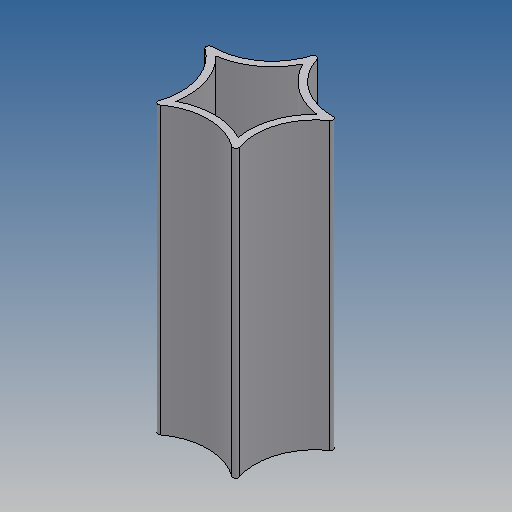
# Autodesk Inventor part: 21700_stern
Saved by Autodesk Inventor 2019.4 (Build 234330000, 330)
## iProperties
Part Number: 21700_stern
Material: GEDA Stahl
Document SubType Name: Modeling
Designer: Admin
Mass: 31.4795 g
Surface Area: 66.7703 cm^2
Volume: 4.00503 cm^3
Density: 7.86 g/cm^3
Appearance: GEDA Stahl A
Gewicht: 0,031 kg
G_L: 0
G_H: 0
G_B: 0
InventorVersion: 2019.4
VAULT_Status: in Bearbeitung
Revision: -
Max. Breite: 0
Max. Höhe: 0
Max. Länge: 0
Max. Abmessungen: 0 x 0 x 0
Volumen: 4005,026
Author: Admin
Autodesk Inventor part; units mm, degrees
note: some values were not read from the file. Left out: dimensions or parameters whose unit could not be read.
ref_plane "YZ Plane" through (0, 0, 0) normal (1, 0, 0) x (0, 1, 0)
ref_plane "XZ Plane" through (0, 0, 0) normal (0, 1, 0) x (-1, 0, 0)
ref_plane "XY Plane" through (0, 0, 0) normal (0, 0, 1) x (1, 0, 0)
sketch "Skizze1" plane through (0, 0, 0) normal (0, 0, 1) x (1, 0, 0)
  circle A0 centre (-10.5, 14.452) radius 10.5
  circle A1 centre (0, 0) radius 17.8637 construction
  circle A2 centre (10.5, 14.452) radius 10.5
  circle A3 centre (16.9894, -5.5202) radius 10.5
  circle A4 centre (0, -17.8637) radius 10.5
  circle A5 centre (-16.9894, -5.5202) radius 10.5
  arc A6 (-13.7447, 4.4659) -> (0, 14.452) centre (-10.5, 14.452) ccw
  arc A7 (0, 14.452) -> (13.7447, 4.4659) centre (10.5, 14.452) ccw
  arc A8 (13.7447, 4.4659) -> (8.4947, -11.6919) centre (16.9894, -5.5202) ccw
  arc A9 (8.4947, -11.6919) -> (-8.4947, -11.6919) centre (0, -17.8637) ccw
  arc A10 (-8.4947, -11.6919) -> (-13.7447, 4.4659) centre (-16.9894, -5.5202) ccw
  dimension "d0" = 21
  dimension "d1" = 10.5
  constraints: 15 point on circle, 13 equal radius, 11 centre point, 6 coincident, 1 vertical alignment
  measures "d0" diameter of A0
  measures "d1" radius of A7
extrude "Extrusion1" add sketch "Skizze1" along normal blind 50 contours A2 A3 A4 A5 A0
fillet "Rundung1" radius 0.5 5 edges at (0, 14.452, 25) (13.7447, 4.4659, 25) (-13.7447, 4.4659, 25) (-8.4947, -11.6919, 25) (8.4947, -11.6919, 25)
sketch "Skizze2" plane through (0, 0, 50) normal (0, 0, 1) x (1, 0, 0)
  arc A0 (6.269, -9.4405) -> (7.0412, -8.8794) centre (6.5675, -9.0394) ccw projected
  arc A1 (10.9157, 3.0449) -> (7.0412, -8.8794) centre (16.9894, -5.5202) ccw projected
  arc A2 (10.9157, 3.0449) -> (10.6207, 3.9527) centre (10.6264, 3.4527) ccw projected
  arc A3 (0.4773, 11.3223) -> (10.6207, 3.9527) centre (10.5, 14.452) ccw projected
  arc A4 (0.4773, 11.3223) -> (-0.4773, 11.3223) centre (0, 11.1733) ccw projected
  arc A5 (-10.6207, 3.9527) -> (-0.4773, 11.3223) centre (-10.5, 14.452) ccw projected
  arc A6 (-10.6207, 3.9527) -> (-10.9157, 3.0449) centre (-10.6264, 3.4527) ccw projected
  arc A7 (-7.0412, -8.8794) -> (-10.9157, 3.0449) centre (-16.9894, -5.5202) ccw projected
  arc A8 (-7.0412, -8.8794) -> (-6.269, -9.4405) centre (-6.5675, -9.0394) ccw projected
  arc A9 (6.269, -9.4405) -> (-6.269, -9.4405) centre (0, -17.8637) ccw projected
  arc A10 (8.8359, 2.871) -> (5.4609, -7.5163) centre (16.9894, -5.5202) ccw
  arc A11 (5.4609, -7.5163) -> (-5.4609, -7.5163) centre (0, -17.8637) ccw
  arc A12 (-5.4609, -7.5163) -> (-8.8359, 2.871) centre (-16.9894, -5.5202) ccw
  arc A13 (-8.8359, 2.871) -> (0, 9.2906) centre (-10.5, 14.452) ccw
  arc A14 (0, 9.2906) -> (8.8359, 2.871) centre (10.5, 14.452) ccw
  point P0 (0, 0)
  dimension "d5" = 1.2
  constraints: 10 point on circle, 5 centre point, 4 other
  measures "d5" radial gap between concentric circles of A3 A14
extrude "Extrusion2" cut sketch "Skizze2" against normal through all contours A10 A11 A12 A13 A14
equation "\"G_L\" = 0"
equation "\"G_H\" = 0"
equation "\"G_B\" = 0"
